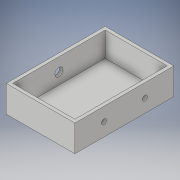
# Autodesk Inventor part: bottom
Saved by Autodesk Inventor 2017 SP1 (Build 210196100, 196)
## iProperties
Created: 2016-12-24
Part Number: bottom
Material: Generic
Document SubType Name: Modeling
Designer: wsh32
Density: 1 g/cm^3
Appearance: Default
Author: wsh32
Autodesk Inventor part; units mm, degrees
ref_plane "YZ Plane" through (0, 0, 0) normal (1, 0, 0) x (0, 1, 0)
ref_plane "XZ Plane" through (0, 0, 0) normal (0, 1, 0) x (-1, 0, 0)
ref_plane "XY Plane" through (0, 0, 0) normal (0, 0, 1) x (1, 0, 0)
sketch "Sketch3" plane through (0, 0, 0) normal (0, 1, 0) x (-1, 0, 0)
  line L0 (0, 0) -> (-106.68, 0)
  line L1 (-106.68, 0) -> (-106.68, -153.67)
  line L2 (-106.68, -153.67) -> (0, -153.67)
  line L3 (0, -153.67) -> (0, 0)
  line L4 (-15.24, -138.43) -> (-91.44, -138.43) construction
  line L5 (-91.44, -138.43) -> (-91.44, -87.63) construction
  line L6 (-91.44, -87.63) -> (-15.24, -87.63) construction
  line L7 (-15.24, -87.63) -> (-15.24, -138.43) construction
  line L8 (-15.24, -66.04) -> (-91.44, -66.04) construction
  line L9 (-91.44, -66.04) -> (-91.44, -15.24) construction
  line L10 (-91.44, -15.24) -> (-15.24, -15.24) construction
  line L11 (-15.24, -15.24) -> (-15.24, -66.04) construction
  dimension "d0" = 76.2
  dimension "d1" = 50.8
  dimension "d2" = 15.24
  dimension "d3" = 15.24
  dimension "d4" = 15.24
  dimension "d5" = 15.24
  dimension "d6" = 21.59
  constraints: 24 end point, 6 parallel, 3 horizontal, 3 perpendicular, 2 equal length, 1 collinear
  measures "d0" distance of L4.start L4.end
  measures "d1" distance of L6.end L4.start
  measures "d2" distance between parallel lines of L3 L7
  measures "d3" distance between parallel lines of L1 L5
  measures "d4" distance between parallel lines of L2 L4
  measures "d5" distance between parallel lines of L0 L10
  measures "d6" distance between parallel lines of L6 L8
extrude "Extrusion1" add sketch "Sketch3" along normal blind 3.175
sketch "Sketch4" plane through (0, 3.175, 0) normal (0, 1, 0) x (1, 0, 0)
  line L0 (0, 0) -> (106.68, 0) projected
  line L1 (106.68, 0) -> (106.68, 153.67) projected
  line L2 (106.68, 153.67) -> (0, 153.67) projected
  line L3 (0, 153.67) -> (0, 0) projected
  line L4 (5.08, 5.08) -> (101.6, 5.08)
  line L5 (101.6, 5.08) -> (101.6, 148.59)
  line L6 (101.6, 148.59) -> (5.08, 148.59)
  line L7 (5.08, 148.59) -> (5.08, 5.08)
  dimension "d9" = 5.08
  constraints: 8 end point, 3 other
  measures "d9" distance between parallel lines of L3 L7
extrude "Extrusion2" add sketch "Sketch4" along normal blind 38.1
sketch "Sketch5" plane through (0, 3.175, 0) normal (0, 1, 0) x (1, 0, 0)
  line L0 (18.9992, 137.8966) -> (87.6808, 137.8966) construction
  line L1 (87.6808, 137.8966) -> (87.6808, 15.7734) construction
  line L2 (87.6808, 15.7734) -> (18.9992, 15.7734) construction
  line L3 (18.9992, 15.7734) -> (18.9992, 137.8966) construction
  line L4 (18.9992, 15.7734) -> (87.6808, 15.7734) construction
  line L5 (87.6808, 15.7734) -> (87.6808, 64.135) construction
  line L6 (87.6808, 64.135) -> (18.9992, 64.135) construction
  line L7 (18.9992, 64.135) -> (18.9992, 15.7734) construction
  line L8 (87.6808, 137.8966) -> (18.9992, 137.8966) construction
  line L9 (18.9992, 137.8966) -> (18.9992, 89.535) construction
  line L10 (18.9992, 89.535) -> (87.6808, 89.535) construction
  line L11 (87.6808, 89.535) -> (87.6808, 137.8966) construction
  line L12 (5.08, 148.59) -> (5.08, 5.08) construction
  line L13 (5.08, 5.08) -> (101.6, 5.08) construction
  line L14 (101.6, 5.08) -> (101.6, 148.59) construction
  line L15 (101.6, 148.59) -> (5.08, 148.59) construction
  point P0 (0, 0)
  dimension "d12" = 68.6816
  dimension "d13" = 48.3616
  dimension "d14" = 48.3616
  dimension "d15" = 13.9192
  dimension "d16" = 10.6934
  dimension "d17" = 10.6934
  dimension "d18" = 13.9192
  dimension "d19" = 25.4
  constraints: 24 end point, 6 parallel, 3 horizontal, 3 perpendicular, 2 point on line
  measures "d12" distance of L1.end L2.end
  measures "d13" distance between parallel lines of L2 L6
  measures "d14" distance between parallel lines of L0 L10
  measures "d15" distance between parallel lines of L12 L3
  measures "d16" distance between parallel lines of L13 L2
  measures "d17" distance between parallel lines of L15 L0
  measures "d18" distance between parallel lines of L14 L1
  measures "d19" distance between parallel lines of L10 L6
sketch "Sketch6" plane through (106.68, 0, 0) normal (1, 0, 0) x (0, 0, -1)
  line L0 (45.085, 20.6375) -> (108.585, 20.6375) construction
  line L1 (0, 41.275) -> (153.67, 41.275) projected
  line L2 (0, 0) -> (153.67, 0) projected
  line L3 (0, 0) -> (0, 41.275) projected
  line L4 (153.67, 0) -> (153.67, 41.275) projected
  dimension "d20" = 20.6375
  dimension "d21" = 20.6375
  dimension "d22" = 45.085
  dimension "d23" = 45.085
  dimension "d24" = 63.5
  constraints: 2 coincident, 2 end point, 1 horizontal
  measures "d20" distance between parallel lines of L1 L0
  measures "d21" distance between parallel lines of L2 L0
  measures "d22" distance from line of L3 L0.start
  measures "d23" distance from line of L4 L0.end
  measures "d24" distance of L0.start L0.end
hole "Hole1" at (106.68, 20.6375, -45.085) at (106.68, 20.6375, -108.585) direction (-1, 0, 0) diameter 7.62 end up to face face through (101.6, 28.575, -52.9167) facing (-1, 0, 0)
sketch "Sketch7" plane through (0, 0, -153.67) normal (-1, 0, 0) x (0, 0, 1)
  line L0 (0, 0) -> (153.67, 0) projected
  line L1 (0, 41.275) -> (153.67, 41.275) projected
  line L2 (153.67, 0) -> (153.67, 41.275) projected
  line L3 (0, 0) -> (0, 41.275) projected
  point P0 (76.835, 20.6375)
  dimension "d32" = 20.6375
  dimension "d33" = 20.6375
  dimension "d34" = 76.835
  dimension "d35" = 76.835
  measures "d32" distance from line of L0 point (76.835, 20.638)
  measures "d33" distance from line of L1 point (76.835, 20.638)
  measures "d34" distance from line of L2 point (76.835, 20.638)
  measures "d35" distance from line of L3 point (76.835, 20.638)
hole "Hole2" at (0, 20.6375, -76.835) direction (1, 0, 0) diameter 12.7 end up to face face through (5.08, 28.575, -100.7533) facing (1, 0, 0)
equation "\"d3\" = d2"
equation "\"d4\" = d2"
equation "\"d5\" = d3"
equation "\"d17\" = d16"
equation "\"d18\" = d15"
equation "\"d20\" = d21"
equation "\"d23\" = d22"
equation "\"d32\" = d33"
equation "\"d34\" = d35"
body "Solid1"
